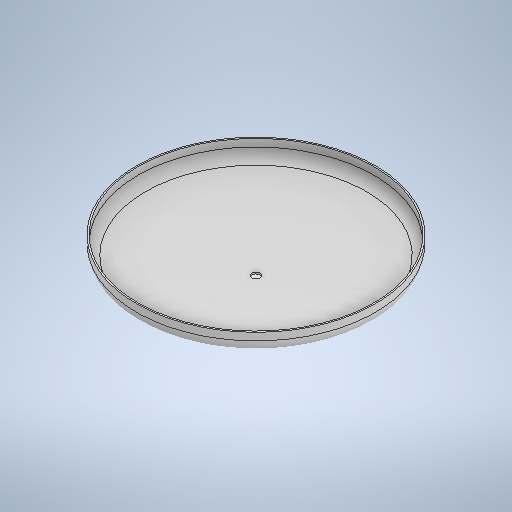
# Autodesk Inventor part: Сферическое дно D1000
Saved by Autodesk Inventor 2025 (Build 290162010, 162A)
## iProperties
Created: 2025-02-16
Part Number: Сферическое дно D1000
Material: Generic
Document SubType Name: Modeling
Designer: pokla
Density: 1 g/cm^3
Appearance: Default
Author: pokla
Autodesk Inventor part; units mm, degrees
ref_plane "YZ Plane" through (0, 0, 0) normal (1, 0, 0) x (0, 1, 0)
ref_plane "XZ Plane" through (0, 0, 0) normal (0, 1, 0) x (-1, 0, 0)
ref_plane "XY Plane" through (0, 0, 0) normal (0, 0, 1) x (1, 0, 0)
sketch "Sketch1" plane through (0, 0, 0) normal (0, 1, 0) x (-1, 0, 0)
  line L0 (480.5, 0) -> (480.5, -30)
  arc A0 (445.9689, -77.547) -> (480.5, -30) centre (430.5, -30) ccw
  arc A1 (0, -148.2683) -> (445.9689, -77.547) centre (0, 1293.2317) ccw
  line L1 (0, 191.6842) -> (0, -191.6842)
  arc A2 (0, -142.2683) -> (444.1126, -71.8413) centre (0, 1293.2317) ccw
  arc A3 (444.1126, -71.8413) -> (474.5, -30) centre (430.5, -30) ccw
  line L2 (474.5, -30) -> (474.5, 0)
  line L3 (474.5, 0) -> (480.5, 0)
  line L4 (0, -142.2683) -> (0, -148.2683)
  point P0 (0, 0)
  point P1 (0, 0)
  point P2 (0, -145.2683)
  dimension "d0" = 50
  dimension "d1" = 30
  dimension "d3" = 1441.5
  dimension "d4" = 480.5
  dimension "d6" = 6
  constraints: 10 end point, 8 point on circle, 4 centre point, 2 midpoint, 2 tangent, 2 vertical, 1 coincident, 1 horizontal, 1 horizontal alignment, 1 line through centre, 1 parallel, 1 vertical alignment, 2 other
  measures "d0" radius of A0
  measures "d1" distance of L0.start L0.end
  measures "d3" radius of A1
  measures "d4" distance of point (0, 0) L0.start
  measures "d6" radial gap between concentric circles of A1 A2
revolve "Revolution1" add sketch "Sketch1" angle 360 about axis through (0, 0, 191.6842) along (0, 0, -1)
sketch "Sketch2" plane through (0, 0, 0) normal (0, 0, 1) x (1, 0, 0)
  circle A0 centre (0, 0) radius 16.75
  dimension "d8" = 33.5
  constraints: 1 centre point, 1 coincident
  measures "d8" diameter of A0
extrude "Extrusion1" cut sketch "Sketch2" against normal through all
body "Solid1"
